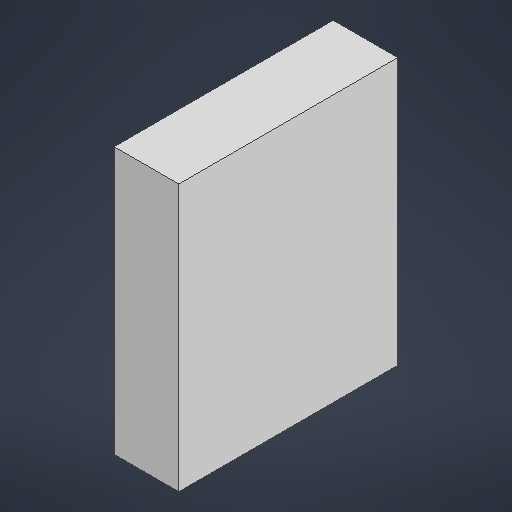
# Autodesk Inventor part: Metal_Bar1
Saved by Autodesk Inventor 2026.2 (Build 302298000, 298)
## iProperties
Created: 2026-07-02
Part Number: Metal_Bar1
Material: Generic
Document SubType Name: Modeling
Designer: usman
Density: 1 g/cm^3
Appearance: Default
Author: usman
Autodesk Inventor part; units mm, degrees
ref_plane "YZ Plane" through (0, 0, 0) normal (1, 0, 0) x (0, 1, 0)
ref_plane "XZ Plane" through (0, 0, 0) normal (0, 1, 0) x (-1, 0, 0)
ref_plane "XY Plane" through (0, 0, 0) normal (0, 0, 1) x (1, 0, 0)
sketch "Sketch1" plane through (0, 0, 0) normal (1, 0, 0) x (0, 1, 0)
  line L0 (38.0137, 56.41) -> (-119.0863, 56.41)
  line L1 (-119.0863, 56.41) -> (-119.0863, -72.69)
  line L2 (-119.0863, -72.69) -> (38.0137, -72.69)
  line L3 (38.0137, -72.69) -> (38.0137, 56.41)
  point P0 (0, 0)
  dimension "d0" = 129.1
  dimension "d1" = 157.1
  constraints: 8 end point, 2 parallel, 1 horizontal, 1 perpendicular
  measures "d0" distance of L2.end L0.start
  measures "d1" distance of L0.start L0.end
extrude "Extrusion1" add sketch "Sketch1" along normal blind 38.1
body "Solid1"
